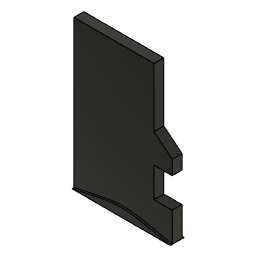
SD卡 v1 v1 (Autodesk Fusion 360 design; units mm, degrees)
Autodesk Fusion 360 part; units mm, degrees
sketch "草图1" plane through (0, 0, 0) normal (0, 1, 0) x (1, 0, 0)
  line L0 (0, 0) -> (10, 0)
  line L1 (8.1421, -15) -> (0, -15)
  line L2 (0, -15) -> (0, 0)
  line L3 (8.1421, -15) -> (8.1421, -9)
  line L4 (8.1421, -9) -> (10, -7.5)
  line L5 (10, -6.0419) -> (8.1421, -6.0419)
  line L6 (8.1421, -6.0419) -> (8.1421, -3)
  line L7 (8.1421, -3) -> (10, -3)
  line L8 (10, 0) -> (10, -3)
  line L9 (10, -6.0419) -> (10, -7.5)
  dimension "d1" = 10
  dimension "d2" = 15
  constraint horizontal L0
  constraint vertical L8
  constraint horizontal L1
  constraint vertical L2
  constraint coincident L0.start L2.end
  constraint perpendicular L1 L3
  constraint coincident L5.start L8
  constraint perpendicular L5 L8
  constraint perpendicular L5 L6
  constraint perpendicular L7 L8
  constraint collinear L8 L9
  measures "d1" distance of L0.start L0.end
  measures "d2" distance of L0.start L1.end
extrude "拉伸1" add sketch "草图1" along normal blind 1
sketch "草图2" plane through (0, 0, 0) normal (0, -1, 0) x (1, 0, 0)
  line L0 (8.1421, 3) -> (8.1421, 6.0419)
  line L1 (8.1421, 6.0419) -> (10, 6.0419)
  line L2 (10, 6.0419) -> (10, 7.5)
  line L3 (10, 7.5) -> (8.1421, 9)
  line L4 (8.1421, 9) -> (8.1421, 15)
  line L5 (8.1421, 15) -> (0, 15)
  line L6 (0, 15) -> (0, 0)
  line L7 (0, 0) -> (10, 0)
  line L8 (10, 0) -> (10, 3)
  line L9 (10, 3) -> (8.1421, 3)
  spline S0 degree 2 poles (0, 0) (5, 1.1516) (10, 0) knots 0 0 0 1.014809 1.014809 1.014809 weights 1 3 1
  constraint coincident L7.end L8.start
  constraint coincident L6.end L7.start
extrude "拉伸2" add sketch "草图2" along normal blind 0.2 contours L7 S0
sketch "草图3" plane through (0, 1, 0) normal (0, 1, 0) x (-1, 0, 0)
  line L0 (-8.1421, 6.0419) -> (-8.1421, 3)
  line L1 (-8.1421, 3) -> (-10, 3)
  line L2 (-10, 3) -> (-10, 0)
  line L3 (-10, 0) -> (0, 0)
  line L4 (0, 0) -> (0, 15)
  line L5 (0, 15) -> (-8.1421, 15)
  line L6 (-8.1421, 15) -> (-8.1421, 9)
  line L7 (-8.1421, 9) -> (-10, 7.5)
  line L8 (-10, 7.5) -> (-10, 6.0419)
  line L9 (-10, 6.0419) -> (-8.1421, 6.0419)
  spline S0 degree 2 poles (-10, 0) (-5, 0.809) (0, 0) knots 0 0 0 1.007336 1.007336 1.007336 weights 1 3 1
  constraint coincident L3.end L4.start
  constraint coincident L2.end L3.start
extrude "拉伸3" add sketch "草图3" along normal blind 0.2 contours L3 S0
